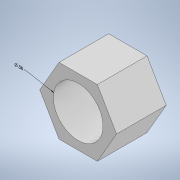
# Autodesk Inventor part: 17mmTo0.5inchBearing
Saved by Autodesk Inventor 2021.2 (Build 252289000, 289)
## iProperties
Created: 2021-03-02
Part Number: 17mmTo0.5inchBearing
Material: Generic
Document SubType Name: Modeling
Designer: robst
Density: 1 g/cm^3
Appearance: Default
Author: robst
Autodesk Inventor part; units mm, degrees
ref_plane "YZ Plane" through (0, 0, 0) normal (1, 0, 0) x (0, 1, 0)
ref_plane "XZ Plane" through (0, 0, 0) normal (0, 1, 0) x (-1, 0, 0)
ref_plane "XY Plane" through (0, 0, 0) normal (0, 0, 1) x (1, 0, 0)
sketch "Sketch1" plane through (0, 0, 0) normal (0, 0, 1) x (1, 0, 0)
  line L0 (4.9075, 8.5) -> (9.815, 0)
  line L1 (9.815, 0) -> (4.9075, -8.5)
  line L2 (4.9075, -8.5) -> (-4.9075, -8.5)
  line L3 (-4.9075, -8.5) -> (-9.815, 0)
  line L4 (-9.815, 0) -> (-4.9075, 8.5)
  line L5 (-4.9075, 8.5) -> (4.9075, 8.5)
  circle A0 centre (0, 0) radius 6.35
  dimension "d0" = 17
  dimension "d1" = 12.7
  constraints: 12 end point, 2 coincident, 1 centre point, 1 horizontal, 13 other
  measures "d0" distance between parallel lines of L2 L5
  measures "d1" diameter of A0
extrude "Extrusion1" add sketch "Sketch1" along normal mid plane 12.7
equation "\"d0\" = hexOutput"
equation "\"d1\" = shaftSize"
equation "\"d2\" = length"
equation "\"hexOutput\" = 17"
equation "\"shaftSize\" = 12.7"
equation "\"length\" = 12.7"
body "Solid1"
